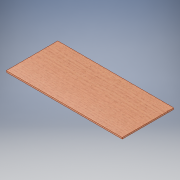
# Autodesk Inventor part: OpticalDeviceRoof
Saved by Autodesk Inventor 2017 (Build 210142000, 142)
## iProperties
Created: 2019-04-10
Part Number: OpticalDeviceRoof
Material: Generic
Document SubType Name: Modeling
Designer: Sharat
Density: 1 g/cm^3
Appearance: White Oak - Natural Medium Gloss
Author: Sharat
Autodesk Inventor part; units mm, degrees
ref_plane "YZ Plane" through (0, 0, 0) normal (1, 0, 0) x (0, 1, 0)
ref_plane "XZ Plane" through (0, 0, 0) normal (0, 1, 0) x (-1, 0, 0)
ref_plane "XY Plane" through (0, 0, 0) normal (0, 0, 1) x (1, 0, 0)
sketch "Sketch1" plane through (0, 0, 0) normal (0, 1, 0) x (-1, 0, 0)
  line L0 (0, 0) -> (-382.9, 0)
  line L1 (-382.9, 0) -> (-382.9, -170)
  line L2 (-382.9, -170) -> (0, -170)
  line L3 (0, -170) -> (0, 0)
  dimension "d0" = 170
  dimension "d1" = 382.9
  constraints: 8 end point, 2 parallel, 1 horizontal, 1 perpendicular
  measures "d0" distance of L0.end L1.end
  measures "d1" distance of L0.start L0.end
extrude "Extrusion1" add sketch "Sketch1" along normal blind 4.7625
body "Solid1"
